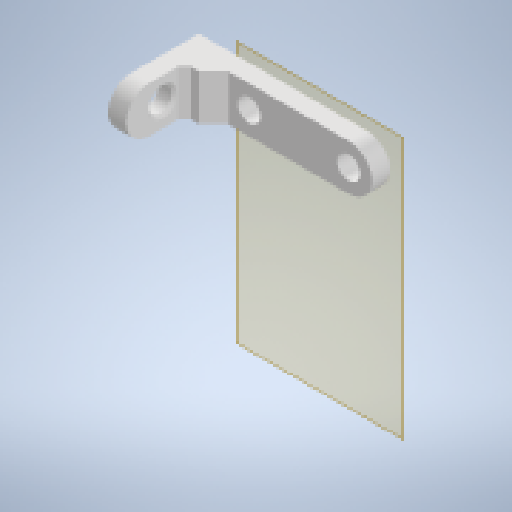
# Autodesk Inventor part: Sensor Mount
Saved by Autodesk Inventor 2024 (Build 280153020, 153B)
## iProperties
Created: 2024-04-02
Part Number: Sensor Mount
Material: Generic
Document SubType Name: Modeling
Designer: lvrectanus0
Density: 1 g/cm^3
Appearance: Default
Author: lvrectanus0
Autodesk Inventor part; units mm, degrees
ref_plane "YZ Plane" through (0, 0, 0) normal (1, 0, 0) x (0, 1, 0)
ref_plane "XZ Plane" through (0, 0, 0) normal (0, 1, 0) x (-1, 0, 0)
ref_plane "XY Plane" through (0, 0, 0) normal (0, 0, 1) x (1, 0, 0)
ref_plane "Work Plane1" through (0, 0, 0) normal (0, 0, 1) x (1, 0, 0)
sketch "Sketch1" plane through (0, 0, 0) normal (0, 0, 1) x (1, 0, 0)
  circle A0 centre (21.4625, 30.925) radius 2 projected
  line L0 (0, 34.925) -> (25.4, 34.925) projected
  line L1 (0, 0) -> (0, 34.925) projected
  line L2 (0, 0) -> (2.54, 0) projected
  arc A1 (2.54, 0) -> (24.765, 0) centre (13.6525, 6.1484) ccw projected
  line L3 (24.765, 0) -> (24.765, 25.2044) projected
  arc A2 (24.765, 25.2044) -> (26.5659, 26.7312) centre (21.4625, 30.925) ccw projected
  spline S0 degree 3 poles (25.4, 34.925) (25.7861, 32.1988) (26.1753, 29.4627) (26.5659, 26.7312) knots -1.120112 -1.120112 -1.120112 -1.120112 -0.293842 -0.293842 -0.293842 -0.293842 projected
  circle A3 centre (4, 30.925) radius 2 projected
  circle A4 centre (21.4625, 30.925) radius 2
  circle A5 centre (21.4625, 30.925) radius 4
  circle A6 centre (4, 30.925) radius 2
  circle A7 centre (4, 30.925) radius 4
  line L4 (21.4625, 34.925) -> (4, 34.925)
  line L5 (4, 34.925) -> (4, 26.925)
  line L6 (4, 26.925) -> (21.4625, 26.925)
  line L7 (21.4625, 26.925) -> (21.4625, 34.925)
  line L8 (-7.9063, 34.925) -> (-7.9063, 26.925)
  line L9 (4, 34.925) -> (-7.9063, 34.925)
  line L10 (4, 26.925) -> (-7.9063, 26.925)
  line L11 (-7.9063, 34.925) -> (-4.7313, 34.925)
  line L12 (-4.7313, 34.925) -> (-4.7313, 26.925)
  line L13 (-4.7313, 26.925) -> (-7.9063, 26.925)
  line L14 (-7.9063, 26.925) -> (-7.9063, 34.925)
  point P0 (-20.6063, 34.925)
  dimension "d0" = 12.7
  dimension "d1" = 3.175
  dimension "d2" = 8
  constraints: 22 end point, 7 horizontal, 4 coincident, 4 parallel, 2 centre point, 2 concentric, 2 perpendicular, 2 point on line, 1 vertical, 1 vertical alignment, 5 other
  measures "d0" distance from line of L8 point (-20.606, 34.925)
  measures "d1" distance of L12.end L13.end
  measures "d2" distance of L8.start L8.end
extrude "Extrusion1" add sketch "Sketch1" along normal blind 3.175 contours A0 L7 | A0 L7 A5 | L7 A0 | A0 L7 A5 | A5 L6 A7 L0 | A7 L1 L0 | L5 A3 A7 | A7 L5 A3 | L10 L1 A7 | L1 L10 L12 L9 | L5 A3 | A3 L5 | L12 L10 L8 L9
sketch "Sketch2" plane through (0, 0, 3.175) normal (0, 0, 1) x (1, 0, 0)
  line L0 (-4.7313, 34.925) -> (-4.7313, 26.925) projected
  line L1 (-7.9063, 34.925) -> (-7.9063, 26.925) projected
  line L2 (4, 26.925) -> (-7.9063, 26.925) projected
  line L3 (4, 34.925) -> (-7.9063, 34.925) projected
  point P0 (0, 0)
extrude "Extrusion2" add sketch "Sketch2" along normal blind 12.7
fillet "Fillet1" radius 3.9878 2 edges at (-6.3188, 34.925, 15.875) (-6.3188, 26.925, 15.875)
sketch "Sketch3" plane through (-4.7313, 26.925, 3.175) normal (1, 0, 0) x (0, 0, -1)
  line L0 (0, 8) -> (0, 0) projected
  point P0 (3.175, -26.925)
  point P1 (-6.35, 4)
  point P2 (0, 4)
  point P3 (0, 4)
  dimension "d8" = 6.35
  constraints: 2 midpoint, 1 horizontal alignment
  measures "d8" distance of point (-6.35, 4) point (0, 4)
hole "Hole1" at (-4.7313, 30.925, 9.525) direction (-1, 0, 0) diameter 4 end through all
chamfer "Chamfer1" distance 0.5 angle 45 2 edges at (-7.9063, 30.925, 11.525) (-4.7313, 30.925, 11.525)
sketch "Sketch4" plane through (-4.7313, 26.925, 3.175) normal (1, 0, 0) x (0, 0, -1)
  line L0 (0, 8) -> (0, 0) projected
  line L1 (0, 0) -> (-8.7122, 0) projected
  line L2 (0, 8) -> (-2.54, 8)
  line L3 (-2.54, 8) -> (-2.54, 0)
  line L4 (-2.54, 0) -> (0, 0)
  line L5 (0, 0) -> (0, 8)
  point P0 (3.175, -26.925)
  dimension "d19" = 2.54
  constraints: 8 end point, 2 parallel, 1 horizontal, 1 perpendicular, 1 point on line
  measures "d19" distance of L4.end L3.end
extrude "Extrusion3" add sketch "Sketch4" along normal blind 2.54
chamfer "Chamfer2" distance 1 angle 45 1 edges at (-4.7313, 30.925, 5.715)
chamfer "Chamfer3" distance 2.54 angle 45 1 edges at (-2.1913, 30.925, 3.175)
sketch "Sketch6" plane through (0, 0, 3.175) normal (0, 0, 1) x (1, 0, 0)
  circle A0 centre (21.4625, 30.925) radius 2 projected
  line L0 (0, 34.925) -> (25.4, 34.925) projected
  line L1 (0, 0) -> (0, 34.925) projected
  line L2 (0, 0) -> (2.54, 0) projected
  arc A1 (2.54, 0) -> (24.765, 0) centre (13.6525, 6.1484) ccw projected
  line L3 (24.765, 0) -> (24.765, 25.2044) projected
  arc A2 (24.765, 25.2044) -> (26.5659, 26.7312) centre (21.4625, 30.925) ccw projected
  spline S0 degree 3 poles (25.4, 34.925) (25.7861, 32.1988) (26.1753, 29.4627) (26.5659, 26.7312) knots -1.120112 -1.120112 -1.120112 -1.120112 -0.293842 -0.293842 -0.293842 -0.293842 projected
  circle A3 centre (4, 30.925) radius 2 projected
  constraints: 2 coincident
hole "Hole2" at (21.4625, 30.925, 3.175) at (4, 30.925, 3.175) direction (0, 0, -1) diameter 4 end through all
body "Solid1"
